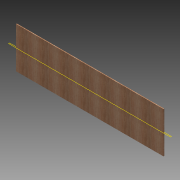
# Autodesk Inventor part: plywood platform
Saved by Autodesk Inventor 2015 (Build 190159000, 159)
## iProperties
Created: 2015-01-03
Part Number: plywood platform
Material: Wood (Birch)
Document SubType Name: Modeling
Designer: Peter
Density: 0.55 g/cm^3
Appearance: Birch - Natural Polished
Author: Peter
Autodesk Inventor part; units mm, degrees
ref_plane "YZ Plane" through (0, 0, 0) normal (1, 0, 0) x (0, 1, 0)
ref_plane "XZ Plane" through (0, 0, 0) normal (0, 1, 0) x (-1, 0, 0)
ref_plane "XY Plane" through (0, 0, 0) normal (0, 0, 1) x (1, 0, 0)
sketch "Sketch1" plane through (0, 0, 0) normal (0, 0, 1) x (1, 0, 0)
  line L0 (0, 0) -> (1828.8, 0)
  line L1 (1828.8, 0) -> (1828.8, 508)
  line L2 (1828.8, 508) -> (0, 508)
  line L3 (0, 508) -> (0, 0)
  dimension "d0" = 1828.8
  dimension "d1" = 508
  constraints: 8 end point, 2 parallel, 1 horizontal, 1 perpendicular
  measures "d0" distance of L2.end L1.end
  measures "d1" distance of L1.end L0.end
extrude "Extrusion1" add sketch "Sketch1" along normal blind 9.525
ref_plane "Work Plane2" through (0, 254, 0) normal (0, 1, 0) x (1, 0, 0)
body "Solid1"
